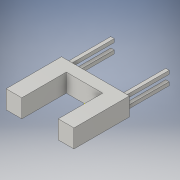
# Autodesk Inventor part: p_inter
Saved by Autodesk Inventor 2016 (Build 200138000, 138)
## iProperties
Created: 2016-02-14
Part Number: p_inter
Material: PC/ABS Plastic
Document SubType Name: Modeling
Designer: jforce
Density: 0.357273 g/cm^3
Appearance: Smooth - White
Author: jforce
Autodesk Inventor part; units mm, degrees
ref_plane "YZ Plane" through (0, 0, 0) normal (1, 0, 0) x (0, 1, 0)
ref_plane "XZ Plane" through (0, 0, 0) normal (0, 1, 0) x (-1, 0, 0)
ref_plane "XY Plane" through (0, 0, 0) normal (0, 0, 1) x (1, 0, 0)
sketch "Sketch1" plane through (0, 0, 0) normal (0, 0, 1) x (1, 0, 0)
  line L0 (-9.3, 0) -> (9.3, 0)
  line L1 (9.3, 0) -> (9.3, 5)
  line L2 (9.3, 5) -> (-9.3, 5)
  line L3 (-9.3, 5) -> (-9.3, 0)
  point P0 (0, 0)
  dimension "d2" = 18.6
  dimension "d3" = 9.3
  dimension "d4" = 5
  dimension "d7" = 0
  constraints: 8 end point, 2 parallel, 1 horizontal, 1 perpendicular
  measures "d2" distance of L1.end L2.end
  measures "d3" distance from line of point (0, 0) L3
  measures "d4" distance of L0.end L1.end
  measures "d7" distance from line of point (0, 0) L0
extrude "Extrusion1" add sketch "Sketch1" along normal blind 3
sketch "Sketch2" plane through (0, 0, 3) normal (0, 0, 1) x (1, 0, 0)
  point P0 (0, 0)
sketch "Sketch3" plane through (0, 0, 3) normal (0, 0, 1) x (1, 0, 0)
  line L0 (9.3, 5) -> (-9.3, 5) projected
  line L1 (-9.3, 0) -> (9.3, 0) projected
  line L2 (-9.3, 5) -> (-5, 5)
  line L3 (-5, 5) -> (-5, 0)
  line L4 (-5, 0) -> (-9.3, 0)
  line L5 (-9.3, 0) -> (-9.3, 5)
  line L6 (0, 0) -> (0, 6.3784) construction
  line L7 (9.3, 5) -> (5, 5)
  line L8 (5, 5) -> (5, 0)
  line L9 (5, 0) -> (9.3, 0)
  line L10 (9.3, 0) -> (9.3, 5)
  point P0 (9.3, 0)
  dimension "d8" = 5
  constraints: 18 end point, 4 symmetric about line, 2 parallel, 1 horizontal, 1 perpendicular, 1 point on line, 1 vertical
  measures "d8" distance from line of L3 L6.start
extrude "Extrusion2" add sketch "Sketch3" along normal blind 12.2 contours L10 L1 L8 L0 | L3 L1 L5 L0
sketch "Sketch4" plane through (0, 0, 0) normal (0, 0, -1) x (-1, 0, 0)
  line L0 (0, 1.1656) -> (-7.6, 1.1656) construction
  line L1 (0, 0) -> (0, 7.9667) construction
  line L2 (-8.0064, 1.6248) -> (-7.0594, 1.6248)
  line L3 (-7.0594, 1.6248) -> (-7.0594, 0.6778)
  line L4 (-7.0594, 0.6778) -> (-8.0064, 0.6778)
  line L5 (-8.0064, 0.6778) -> (-8.0064, 1.6248)
  line L6 (-9.3, 0) -> (-9.3, 5) projected
  line L7 (-9.3, 2.5) -> (9.3, 2.5) construction
  line L8 (9.3, 5) -> (9.3, 0) projected
  line L9 (-8.0064, 3.3752) -> (-7.0594, 3.3752)
  line L10 (-7.0594, 3.3752) -> (-7.0594, 4.3222)
  line L11 (-7.0594, 4.3222) -> (-8.0064, 4.3222)
  line L12 (-8.0064, 4.3222) -> (-8.0064, 3.3752)
  line L13 (8.0064, 1.6248) -> (7.0594, 1.6248)
  line L14 (7.0594, 1.6248) -> (7.0594, 0.6778)
  line L15 (7.0594, 0.6778) -> (8.0064, 0.6778)
  line L16 (8.0064, 0.6778) -> (8.0064, 1.6248)
  line L17 (8.0064, 3.3752) -> (7.0594, 3.3752)
  line L18 (7.0594, 3.3752) -> (7.0594, 4.3222)
  line L19 (7.0594, 4.3222) -> (8.0064, 4.3222)
  line L20 (8.0064, 4.3222) -> (8.0064, 3.3752)
  dimension "d11" = 7.6
  constraints: 38 end point, 12 symmetric about line, 2 midpoint, 2 parallel, 1 horizontal, 1 perpendicular, 1 vertical
  measures "d11" distance of L0.start L0.end
extrude "Extrusion3" add sketch "Sketch4" along normal blind 12.2
body "Solid1"
